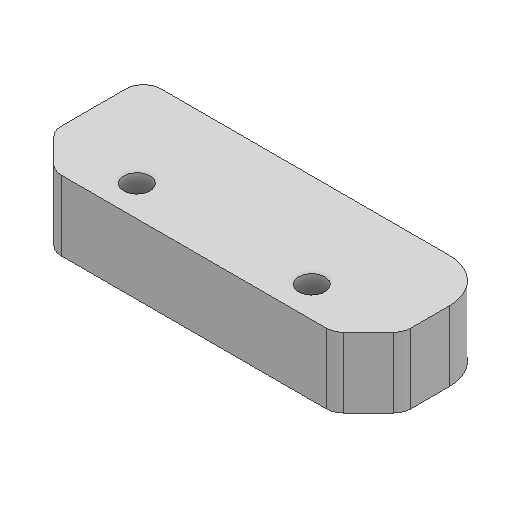
# Autodesk Inventor part: 3DP_ABS_Y_Axis_Cable_Chain_Mounting_Bracket
Saved by Autodesk Inventor 2026.1 (Build 301233000, 233)
## iProperties
Created: 2016-06-22
Part Number: 3DP_ABS_Y_Axis_Cable_Chain_Mounting_Bracket
Material: Ogólny
Document SubType Name: Modeling
Designer: Andrzej
Density: 1 g/cm^3
Appearance: Domyślna
Mass: 4.31615 g
Surface Area: 20.5759 cm^2
Volume: 4.31615 cm^3
Author: Andrzej
Autodesk Inventor part; units mm, degrees
ref_plane "YZ Plane" through (0, 0, 0) normal (1, 0, 0) x (0, 1, 0)
ref_plane "XZ Plane" through (0, 0, 0) normal (0, 1, 0) x (-1, 0, 0)
ref_plane "XY Plane" through (0, 0, 0) normal (0, 0, 1) x (1, 0, 0)
sketch "Szkic1" plane through (0, 0, 0) normal (0, 0, 1) x (1, 0, 0)
  line L0 (-7.4523, 3.0496) -> (32.5477, 3.0496)
  line L1 (32.5477, 3.0496) -> (32.5477, -11.2004)
  line L2 (32.5477, -11.2004) -> (-7.4523, -11.2004)
  line L3 (-7.4523, -11.2004) -> (-7.4523, 3.0496)
  point P0 (0, 0)
  point P1 (2.5477, -7.7004)
  point P2 (22.5477, -7.7004)
  dimension "d0" = 40
  dimension "d1" = 14.25
  dimension "d2" = 3.5
  dimension "d3" = 3.5
  dimension "d4" = 10
  dimension "d5" = 10
  constraints: 8 end point, 2 parallel, 1 horizontal, 1 perpendicular
  measures "d0" distance of L1.end L2.end
  measures "d1" distance of L0.end L1.end
  measures "d2" distance from line of L2 point (2.548, -7.7)
  measures "d3" distance from line of L2 point (22.548, -7.7)
  measures "d4" distance from line of L3 point (2.548, -7.7)
  measures "d5" distance from line of L1 point (22.548, -7.7)
extrude "Wyciągnięcie proste1" add sketch "Szkic1" along normal blind 8
hole "Otwór1" at (2.5477, -7.7004, 0) at (22.5477, -7.7004, 0) direction (0, 0, 1) diameter 3 end through all
chamfer "Faza1" distance 4 angle 45 2 edges at (-7.4523, -11.2004, 4) (32.5477, -11.2004, 4)
fillet "Zaokrąglenie1" radius 2 4 edges at (32.5477, -7.2004, 4) (28.5477, -11.2004, 4) (-3.4523, -11.2004, 4) (-7.4523, -7.2004, 4)
fillet "Zaokrąglenie4" radius 5 1 edges at (32.5477, 3.0496, 4)
fillet "Zaokrąglenie5" radius 2 1 edges at (-7.4523, 3.0496, 4)
